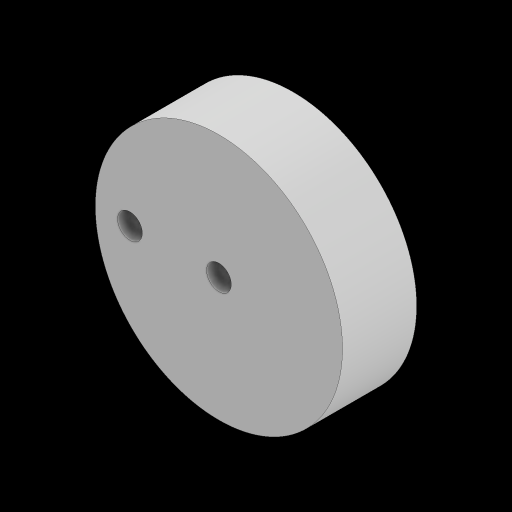
# Autodesk Inventor part: SC-1-01-Capper train
Saved by Autodesk Inventor 2023 (Build 270158000, 158)
## iProperties
Created: 2023-01-30
Part Number: SC-1-01-Capper train
Material: Generic
Document SubType Name: Modeling
Designer: annah
Density: 1 g/cm^3
Appearance: Default
Author: annah
Autodesk Inventor part; units mm, degrees
ref_plane "YZ Plane" through (0, 0, 0) normal (1, 0, 0) x (0, 1, 0)
ref_plane "XZ Plane" through (0, 0, 0) normal (0, 1, 0) x (-1, 0, 0)
ref_plane "XY Plane" through (0, 0, 0) normal (0, 0, 1) x (1, 0, 0)
sketch "Sketch1" plane through (0, 0, 0) normal (0, 0, 1) x (1, 0, 0)
  circle A0 centre (0, 0) radius 25
  circle A1 centre (0, 0) radius 2.5
  circle A2 centre (-18, 0) radius 2.5
  dimension "d0" = 50
  dimension "d1" = 5
  dimension "d4" = 5
  dimension "d5" = 18
  constraints: 3 centre point, 2 coincident
  measures "d0" diameter of A0
  measures "d1" diameter of A1
  measures "d4" diameter of A2
  measures "d5" distance of A2.centre point (0, 0)
extrude "Extrusion1" add sketch "Sketch1" along normal blind 15
body "Solid1"
